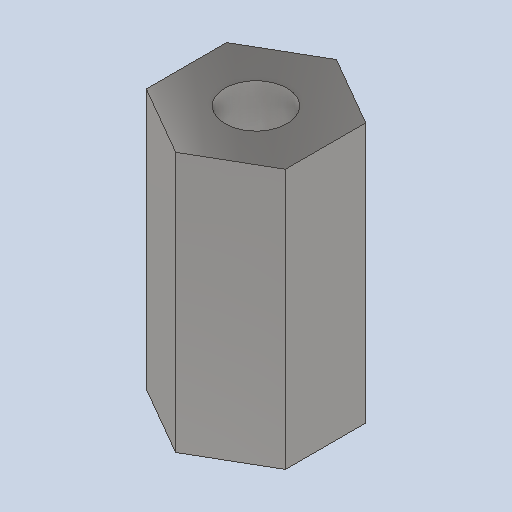
# Autodesk Inventor part: pc104standoffTEMP2
Saved by Autodesk Inventor 2022 (Build 260153000, 153)
## iProperties
Created: 2021-04-30
Part Number: pc104standoffTEMP2
Material: Stainless Steel
Document SubType Name: Modeling
Designer: Bowen O'Steen
Density: 8 g/cm^3
Appearance: Semi-Polished
Author: Bowen O'Steen
Autodesk Inventor part; units mm, degrees
ref_plane "YZ Plane" through (0, 0, 0) normal (1, 0, 0) x (0, 1, 0)
ref_plane "XZ Plane" through (0, 0, 0) normal (0, 1, 0) x (-1, 0, 0)
ref_plane "XY Plane" through (0, 0, 0) normal (0, 0, 1) x (1, 0, 0)
sketch "Sketch1" plane through (0, 0, 0) normal (0, 1, 0) x (-1, 0, 0)
  line L0 (3.2, 1.8475) -> (3.2, -1.8475)
  line L1 (3.2, -1.8475) -> (0, -3.695)
  line L2 (0, -3.695) -> (-3.2, -1.8475)
  line L3 (-3.2, -1.8475) -> (-3.2, 1.8475)
  line L4 (-3.2, 1.8475) -> (0, 3.695)
  line L5 (0, 3.695) -> (3.2, 1.8475)
  point P0 (0, 0)
  point P1 (3.2, 0)
  point P2 (-3.2, 0)
  dimension "d0" = 6.4
  dimension "d1" = 120
  dimension "d2" = 6.4
  constraints: 12 end point, 4 parallel, 2 horizontal alignment, 2 midpoint, 2 vertical alignment, 1 vertical
  measures "d0" distance between parallel lines of L3 L0
  measures "d1" angle of L5 L4
  measures "d2" distance between parallel lines of L2 L5
extrude "Extrusion1" add sketch "Sketch1" along normal blind 11.96
sketch "Sketch3" plane through (0, 0, 0) normal (0, -1, 0) x (1, 0, 0)
  circle A0 centre (0, 0) radius 1.4224
  dimension "d8" = 2.8448
  constraints: 1 centre point, 1 coincident
  measures "d8" diameter of A0
extrude "Extrusion3" cut sketch "Sketch3" against normal through all
body "Solid1"
